Autodesk Inventor part; units mm, degrees
(part 2 of 3)
sketch "Sketch8" plane through (0, 0, 9) normal (0, 0, -1) x (-1, 0, 0)
  circle A0 centre (-7.891, 75.5745) radius 2.55 projected
  circle A1 centre (-45.291, 75.5745) radius 2.55 projected
  circle A2 centre (-26.591, 75.5745) radius 2.55 projected
  arc A3 (-14.3665, 90.3518) -> (-12.2661, 92.5181) centre (-15.59, 93.6395) ccw projected
  arc A4 (-14.955, 86.1645) -> (-14.3665, 90.3518) centre (-14.955, 88.2995) ccw projected
  line L0 (-17.86, 86.1645) -> (-14.955, 86.1645) projected
  line L1 (-17.86, 86.6645) -> (-17.86, 86.1645) projected
  line L2 (-14.955, 86.6645) -> (-17.86, 86.6645) projected
  arc A5 (-14.955, 86.6645) -> (-14.955, 89.9345) centre (-14.955, 88.2995) ccw projected
  line L3 (-16.225, 89.9345) -> (-14.955, 89.9345) projected
  arc A6 (-16.7766, 90.8841) -> (-16.225, 89.9345) centre (-16.225, 90.5695) ccw projected
  arc A7 (-16.7766, 90.8841) -> (-12.6611, 92.9903) centre (-15.59, 93.6395) ccw projected
  arc A8 (-12.6611, 92.9903) -> (-11.1978, 95.4421) centre (-12.6138, 94.6246) ccw projected
  line L4 (-11.8328, 96.5419) -> (-11.1978, 95.4421) projected
  arc A9 (-10.733, 97.1769) -> (-11.8328, 96.5419) centre (-11.2829, 96.8594) ccw projected
  line L5 (-9.2805, 94.6611) -> (-10.733, 97.1769) projected
  line L6 (-9.7135, 94.4111) -> (-9.2805, 94.6611) projected
  line L7 (-11.157, 93.0638) -> (-9.7135, 94.4111) projected
  arc A10 (-12.2661, 92.5181) -> (-11.157, 93.0638) centre (-12.6138, 94.6246) ccw projected
  arc A11 (-19.049, 94.2238) -> (-18.2231, 91.3216) centre (-15.59, 93.6395) ccw projected
  arc A12 (-22.3811, 96.8271) -> (-19.049, 94.2238) centre (-20.5321, 95.7596) ccw projected
  line L8 (-20.9286, 99.3429) -> (-22.3811, 96.8271) projected
  line L9 (-20.4955, 99.0929) -> (-20.9286, 99.3429) projected
  line L10 (-21.948, 96.5771) -> (-20.4955, 99.0929) projected
  arc A13 (-21.948, 96.5771) -> (-19.1161, 94.9421) centre (-20.5321, 95.7596) ccw projected
  line L11 (-18.4811, 96.0419) -> (-19.1161, 94.9421) projected
  arc A14 (-17.3829, 96.0448) -> (-18.4811, 96.0419) centre (-17.9312, 95.7244) ccw projected
  arc A15 (-17.3829, 96.0448) -> (-17.6167, 91.4276) centre (-15.59, 93.6395) ccw projected
  arc A16 (-17.6167, 91.4276) -> (-16.225, 88.9345) centre (-16.225, 90.5695) ccw projected
  line L12 (-14.955, 88.9345) -> (-16.225, 88.9345) projected
  arc A17 (-14.955, 87.6645) -> (-14.955, 88.9345) centre (-14.955, 88.2995) ccw projected
  line L13 (-17.86, 87.6645) -> (-14.955, 87.6645) projected
  line L14 (-17.86, 88.1645) -> (-17.86, 87.6645) projected
  line L15 (-18.3051, 90.0883) -> (-17.86, 88.1645) projected
  arc A18 (-18.2231, 91.3216) -> (-18.3051, 90.0883) centre (-16.225, 90.5695) ccw projected
  arc A19 (-13.3545, 96.3429) -> (-16.2808, 97.0788) centre (-15.59, 93.6395) ccw projected
  arc A20 (-9.4339, 97.9269) -> (-13.3545, 96.3429) centre (-11.2829, 96.8594) ccw projected
  line L16 (-7.9814, 95.4111) -> (-9.4339, 97.9269) projected
  line L17 (-8.4145, 95.1611) -> (-7.9814, 95.4111) projected
  line L18 (-9.867, 97.6769) -> (-8.4145, 95.1611) projected
  arc A21 (-9.867, 97.6769) -> (-12.6989, 96.0419) centre (-11.2829, 96.8594) ccw projected
  line L19 (-12.0639, 94.9421) -> (-12.6989, 96.0419) projected
  arc A22 (-12.6105, 93.9896) -> (-12.0639, 94.9421) centre (-12.6138, 94.6246) ccw projected
  arc A23 (-12.6105, 93.9896) -> (-16.4922, 96.5006) centre (-15.59, 93.6395) ccw projected
  arc A24 (-16.4922, 96.5006) -> (-19.3472, 96.5419) centre (-17.9312, 95.7244) ccw projected
  line L20 (-19.9822, 95.4421) -> (-19.3472, 96.5419) projected
  arc A25 (-21.082, 96.0771) -> (-19.9822, 95.4421) centre (-20.5321, 95.7596) ccw projected
  line L21 (-19.6295, 98.5929) -> (-21.082, 96.0771) projected
  line L22 (-19.1965, 98.3429) -> (-19.6295, 98.5929) projected
  line L23 (-17.3079, 97.7664) -> (-19.1965, 98.3429) projected
  arc A26 (-16.2808, 97.0788) -> (-17.3079, 97.7664) centre (-17.9312, 95.7244) ccw projected
  arc A27 (-33.0665, 90.3518) -> (-30.9661, 92.5181) centre (-34.29, 93.6395) ccw projected
  arc A28 (-33.655, 86.1645) -> (-33.0665, 90.3518) centre (-33.655, 88.2995) ccw projected
  line L24 (-36.56, 86.1645) -> (-33.655, 86.1645) projected
  line L25 (-36.56, 86.6645) -> (-36.56, 86.1645) projected
  line L26 (-33.655, 86.6645) -> (-36.56, 86.6645) projected
  arc A29 (-33.655, 86.6645) -> (-33.655, 89.9345) centre (-33.655, 88.2995) ccw projected
  line L27 (-34.925, 89.9345) -> (-33.655, 89.9345) projected
  arc A30 (-35.4766, 90.8841) -> (-34.925, 89.9345) centre (-34.925, 90.5695) ccw projected
  arc A31 (-35.4766, 90.8841) -> (-31.3611, 92.9903) centre (-34.29, 93.6395) ccw projected
  arc A32 (-31.3611, 92.9903) -> (-29.8978, 95.4421) centre (-31.3138, 94.6246) ccw projected
  line L28 (-30.5328, 96.5419) -> (-29.8978, 95.4421) projected
  arc A33 (-29.433, 97.1769) -> (-30.5328, 96.5419) centre (-29.9829, 96.8594) ccw projected
  line L29 (-27.9805, 94.6611) -> (-29.433, 97.1769) projected
  line L30 (-28.4135, 94.4111) -> (-27.9805, 94.6611) projected
  line L31 (-29.857, 93.0638) -> (-28.4135, 94.4111) projected
  arc A34 (-30.9661, 92.5181) -> (-29.857, 93.0638) centre (-31.3138, 94.6246) ccw projected
  arc A35 (-37.749, 94.2238) -> (-36.9231, 91.3216) centre (-34.29, 93.6395) ccw projected
  arc A36 (-41.0811, 96.8271) -> (-37.749, 94.2238) centre (-39.2321, 95.7596) ccw projected
  line L32 (-39.6286, 99.3429) -> (-41.0811, 96.8271) projected
  line L33 (-39.1955, 99.0929) -> (-39.6286, 99.3429) projected
  line L34 (-40.648, 96.5771) -> (-39.1955, 99.0929) projected
  arc A37 (-40.648, 96.5771) -> (-37.8161, 94.9421) centre (-39.2321, 95.7596) ccw projected
  line L35 (-37.1811, 96.0419) -> (-37.8161, 94.9421) projected
  arc A38 (-36.0829, 96.0448) -> (-37.1811, 96.0419) centre (-36.6312, 95.7244) ccw projected
  arc A39 (-36.0829, 96.0448) -> (-36.3167, 91.4276) centre (-34.29, 93.6395) ccw projected
  arc A40 (-36.3167, 91.4276) -> (-34.925, 88.9345) centre (-34.925, 90.5695) ccw projected
  line L36 (-33.655, 88.9345) -> (-34.925, 88.9345) projected
  arc A41 (-33.655, 87.6645) -> (-33.655, 88.9345) centre (-33.655, 88.2995) ccw projected
  line L37 (-36.56, 87.6645) -> (-33.655, 87.6645) projected
  line L38 (-36.56, 88.1645) -> (-36.56, 87.6645) projected
  line L39 (-37.0051, 90.0883) -> (-36.56, 88.1645) projected
  arc A42 (-36.9231, 91.3216) -> (-37.0051, 90.0883) centre (-34.925, 90.5695) ccw projected
  arc A43 (-32.0545, 96.3429) -> (-34.9808, 97.0788) centre (-34.29, 93.6395) ccw projected
  arc A44 (-28.1339, 97.9269) -> (-32.0545, 96.3429) centre (-29.9829, 96.8594) ccw projected
  line L40 (-26.6814, 95.4111) -> (-28.1339, 97.9269) projected
  line L41 (-27.1145, 95.1611) -> (-26.6814, 95.4111) projected
  line L42 (-28.567, 97.6769) -> (-27.1145, 95.1611) projected
  arc A45 (-28.567, 97.6769) -> (-31.3989, 96.0419) centre (-29.9829, 96.8594) ccw projected
  line L43 (-30.7639, 94.9421) -> (-31.3989, 96.0419) projected
  arc A46 (-31.3105, 93.9896) -> (-30.7639, 94.9421) centre (-31.3138, 94.6246) ccw projected
  arc A47 (-31.3105, 93.9896) -> (-35.1922, 96.5006) centre (-34.29, 93.6395) ccw projected
  arc A48 (-35.1922, 96.5006) -> (-38.0472, 96.5419) centre (-36.6312, 95.7244) ccw projected
  line L44 (-38.6822, 95.4421) -> (-38.0472, 96.5419) projected
  arc A49 (-39.782, 96.0771) -> (-38.6822, 95.4421) centre (-39.2321, 95.7596) ccw projected
  line L45 (-38.3295, 98.5929) -> (-39.782, 96.0771) projected
  line L46 (-37.8965, 98.3429) -> (-38.3295, 98.5929) projected
  line L47 (-36.0079, 97.7664) -> (-37.8965, 98.3429) projected
  arc A50 (-34.9808, 97.0788) -> (-36.0079, 97.7664) centre (-36.6312, 95.7244) ccw projected
  arc A51 (-51.7665, 90.3518) -> (-49.6661, 92.5181) centre (-52.99, 93.6395) ccw projected
  arc A52 (-52.355, 86.1645) -> (-51.7665, 90.3518) centre (-52.355, 88.2995) ccw projected
  line L48 (-55.26, 86.1645) -> (-52.355, 86.1645) projected
  line L49 (-55.26, 86.6645) -> (-55.26, 86.1645) projected
  line L50 (-52.355, 86.6645) -> (-55.26, 86.6645) projected
  arc A53 (-52.355, 86.6645) -> (-52.355, 89.9345) centre (-52.355, 88.2995) ccw projected
  line L51 (-53.625, 89.9345) -> (-52.355, 89.9345) projected
  arc A54 (-54.1766, 90.8841) -> (-53.625, 89.9345) centre (-53.625, 90.5695) ccw projected
  arc A55 (-54.1766, 90.8841) -> (-50.0611, 92.9903) centre (-52.99, 93.6395) ccw projected
  arc A56 (-50.0611, 92.9903) -> (-48.5978, 95.4421) centre (-50.0138, 94.6246) ccw projected
  line L52 (-49.2328, 96.5419) -> (-48.5978, 95.4421) projected
  arc A57 (-48.133, 97.1769) -> (-49.2328, 96.5419) centre (-48.6829, 96.8594) ccw projected
  line L53 (-46.6805, 94.6611) -> (-48.133, 97.1769) projected
  line L54 (-47.1135, 94.4111) -> (-46.6805, 94.6611) projected
  line L55 (-48.557, 93.0638) -> (-47.1135, 94.4111) projected
  arc A58 (-49.6661, 92.5181) -> (-48.557, 93.0638) centre (-50.0138, 94.6246) ccw projected
  arc A59 (-56.449, 94.2238) -> (-55.6231, 91.3216) centre (-52.99, 93.6395) ccw projected
  arc A60 (-59.7811, 96.8271) -> (-56.449, 94.2238) centre (-57.9321, 95.7596) ccw projected
  line L56 (-58.3286, 99.3429) -> (-59.7811, 96.8271) projected
  line L57 (-57.8955, 99.0929) -> (-58.3286, 99.3429) projected
  line L58 (-59.348, 96.5771) -> (-57.8955, 99.0929) projected
  arc A61 (-59.348, 96.5771) -> (-56.5161, 94.9421) centre (-57.9321, 95.7596) ccw projected
  line L59 (-55.8811, 96.0419) -> (-56.5161, 94.9421) projected
  arc A62 (-54.7829, 96.0448) -> (-55.8811, 96.0419) centre (-55.3312, 95.7244) ccw projected
  arc A63 (-54.7829, 96.0448) -> (-55.0167, 91.4276) centre (-52.99, 93.6395) ccw projected
  arc A64 (-55.0167, 91.4276) -> (-53.625, 88.9345) centre (-53.625, 90.5695) ccw projected
  line L60 (-52.355, 88.9345) -> (-53.625, 88.9345) projected
  arc A65 (-52.355, 87.6645) -> (-52.355, 88.9345) centre (-52.355, 88.2995) ccw projected
  line L61 (-55.26, 87.6645) -> (-52.355, 87.6645) projected
  line L62 (-55.26, 88.1645) -> (-55.26, 87.6645) projected
  line L63 (-55.7051, 90.0883) -> (-55.26, 88.1645) projected
  arc A66 (-55.6231, 91.3216) -> (-55.7051, 90.0883) centre (-53.625, 90.5695) ccw projected
  arc A67 (-50.7545, 96.3429) -> (-53.6808, 97.0788) centre (-52.99, 93.6395) ccw projected
  arc A68 (-46.8339, 97.9269) -> (-50.7545, 96.3429) centre (-48.6829, 96.8594) ccw projected
  line L64 (-45.3814, 95.4111) -> (-46.8339, 97.9269) projected
  line L65 (-45.8145, 95.1611) -> (-45.3814, 95.4111) projected
  line L66 (-47.267, 97.6769) -> (-45.8145, 95.1611) projected
  arc A69 (-47.267, 97.6769) -> (-50.0989, 96.0419) centre (-48.6829, 96.8594) ccw projected
  line L67 (-49.4639, 94.9421) -> (-50.0989, 96.0419) projected
  arc A70 (-50.0105, 93.9896) -> (-49.4639, 94.9421) centre (-50.0138, 94.6246) ccw projected
  arc A71 (-50.0105, 93.9896) -> (-53.8922, 96.5006) centre (-52.99, 93.6395) ccw projected
  arc A72 (-53.8922, 96.5006) -> (-56.7472, 96.5419) centre (-55.3312, 95.7244) ccw projected
  line L68 (-57.3822, 95.4421) -> (-56.7472, 96.5419) projected
  arc A73 (-58.482, 96.0771) -> (-57.3822, 95.4421) centre (-57.9321, 95.7596) ccw projected
  line L69 (-57.0295, 98.5929) -> (-58.482, 96.0771) projected
  line L70 (-56.5965, 98.3429) -> (-57.0295, 98.5929) projected
  line L71 (-54.7079, 97.7664) -> (-56.5965, 98.3429) projected
  arc A74 (-53.6808, 97.0788) -> (-54.7079, 97.7664) centre (-55.3312, 95.7244) ccw projected
  arc A75 (-14.3665, 76.7318) -> (-12.2661, 78.8981) centre (-15.59, 80.0195) ccw projected
  arc A76 (-14.955, 72.5445) -> (-14.3665, 76.7318) centre (-14.955, 74.6795) ccw projected
  line L72 (-17.86, 72.5445) -> (-14.955, 72.5445) projected
  line L73 (-17.86, 73.0445) -> (-17.86, 72.5445) projected
  line L74 (-14.955, 73.0445) -> (-17.86, 73.0445) projected
  arc A77 (-14.955, 73.0445) -> (-14.955, 76.3145) centre (-14.955, 74.6795) ccw projected
  line L75 (-16.225, 76.3145) -> (-14.955, 76.3145) projected
  arc A78 (-16.7766, 77.2641) -> (-16.225, 76.3145) centre (-16.225, 76.9495) ccw projected
  arc A79 (-16.7766, 77.2641) -> (-12.6611, 79.3703) centre (-15.59, 80.0195) ccw projected
  arc A80 (-12.6611, 79.3703) -> (-11.1978, 81.8221) centre (-12.6138, 81.0046) ccw projected
  line L76 (-11.8328, 82.9219) -> (-11.1978, 81.8221) projected
  arc A81 (-10.733, 83.5569) -> (-11.8328, 82.9219) centre (-11.2829, 83.2394) ccw projected
  line L77 (-9.2805, 81.0411) -> (-10.733, 83.5569) projected
  line L78 (-9.7135, 80.7911) -> (-9.2805, 81.0411) projected
  line L79 (-11.157, 79.4438) -> (-9.7135, 80.7911) projected
  arc A82 (-12.2661, 78.8981) -> (-11.157, 79.4438) centre (-12.6138, 81.0046) ccw projected
  arc A83 (-19.049, 80.6038) -> (-18.2231, 77.7016) centre (-15.59, 80.0195) ccw projected
  arc A84 (-22.3811, 83.2071) -> (-19.049, 80.6038) centre (-20.5321, 82.1396) ccw projected
  line L80 (-20.9286, 85.7229) -> (-22.3811, 83.2071) projected
  line L81 (-20.4955, 85.4729) -> (-20.9286, 85.7229) projected
  line L82 (-21.948, 82.9571) -> (-20.4955, 85.4729) projected
  arc A85 (-21.948, 82.9571) -> (-19.1161, 81.3221) centre (-20.5321, 82.1396) ccw projected
  line L83 (-18.4811, 82.4219) -> (-19.1161, 81.3221) projected
  arc A86 (-17.3829, 82.4248) -> (-18.4811, 82.4219) centre (-17.9312, 82.1044) ccw projected
  arc A87 (-17.3829, 82.4248) -> (-17.6167, 77.8076) centre (-15.59, 80.0195) ccw projected
  arc A88 (-17.6167, 77.8076) -> (-16.225, 75.3145) centre (-16.225, 76.9495) ccw projected
  line L84 (-14.955, 75.3145) -> (-16.225, 75.3145) projected
  arc A89 (-14.955, 74.0445) -> (-14.955, 75.3145) centre (-14.955, 74.6795) ccw projected
  line L85 (-17.86, 74.0445) -> (-14.955, 74.0445) projected
  line L86 (-17.86, 74.5445) -> (-17.86, 74.0445) projected
  line L87 (-18.3051, 76.4683) -> (-17.86, 74.5445) projected
  arc A90 (-18.2231, 77.7016) -> (-18.3051, 76.4683) centre (-16.225, 76.9495) ccw projected
  arc A91 (-13.3545, 82.7229) -> (-16.2808, 83.4588) centre (-15.59, 80.0195) ccw projected
  arc A92 (-9.4339, 84.3069) -> (-13.3545, 82.7229) centre (-11.2829, 83.2394) ccw projected
  line L88 (-7.9814, 81.7911) -> (-9.4339, 84.3069) projected
  line L89 (-8.4145, 81.5411) -> (-7.9814, 81.7911) projected
  line L90 (-9.867, 84.0569) -> (-8.4145, 81.5411) projected
  arc A93 (-9.867, 84.0569) -> (-12.6989, 82.4219) centre (-11.2829, 83.2394) ccw projected
  line L91 (-12.0639, 81.3221) -> (-12.6989, 82.4219) projected
  arc A94 (-12.6105, 80.3696) -> (-12.0639, 81.3221) centre (-12.6138, 81.0046) ccw projected
  arc A95 (-12.6105, 80.3696) -> (-16.4922, 82.8806) centre (-15.59, 80.0195) ccw projected
  arc A96 (-16.4922, 82.8806) -> (-19.3472, 82.9219) centre (-17.9312, 82.1044) ccw projected
  line L92 (-19.9822, 81.8221) -> (-19.3472, 82.9219) projected
  arc A97 (-21.082, 82.4571) -> (-19.9822, 81.8221) centre (-20.5321, 82.1396) ccw projected
  line L93 (-19.6295, 84.9729) -> (-21.082, 82.4571) projected
  line L94 (-19.1965, 84.7229) -> (-19.6295, 84.9729) projected
  line L95 (-17.3079, 84.1464) -> (-19.1965, 84.7229) projected
  arc A98 (-16.2808, 83.4588) -> (-17.3079, 84.1464) centre (-17.9312, 82.1044) ccw projected
  arc A99 (-33.0665, 76.7318) -> (-30.9661, 78.8981) centre (-34.29, 80.0195) ccw projected
  arc A100 (-33.655, 72.5445) -> (-33.0665, 76.7318) centre (-33.655, 74.6795) ccw projected
  line L96 (-36.56, 72.5445) -> (-33.655, 72.5445) projected
  line L97 (-36.56, 73.0445) -> (-36.56, 72.5445) projected
  line L98 (-33.655, 73.0445) -> (-36.56, 73.0445) projected
  arc A101 (-33.655, 73.0445) -> (-33.655, 76.3145) centre (-33.655, 74.6795) ccw projected
  line L99 (-34.925, 76.3145) -> (-33.655, 76.3145) projected
  arc A102 (-35.4766, 77.2641) -> (-34.925, 76.3145) centre (-34.925, 76.9495) ccw projected
  arc A103 (-35.4766, 77.2641) -> (-31.3611, 79.3703) centre (-34.29, 80.0195) ccw projected
  arc A104 (-31.3611, 79.3703) -> (-29.8978, 81.8221) centre (-31.3138, 81.0046) ccw projected
  line L100 (-30.5328, 82.9219) -> (-29.8978, 81.8221) projected
  arc A105 (-29.433, 83.5569) -> (-30.5328, 82.9219) centre (-29.9829, 83.2394) ccw projected
  line L101 (-27.9805, 81.0411) -> (-29.433, 83.5569) projected
  line L102 (-28.4135, 80.7911) -> (-27.9805, 81.0411) projected
  line L103 (-29.857, 79.4438) -> (-28.4135, 80.7911) projected
  arc A106 (-30.9661, 78.8981) -> (-29.857, 79.4438) centre (-31.3138, 81.0046) ccw projected
  arc A107 (-37.749, 80.6038) -> (-36.9231, 77.7016) centre (-34.29, 80.0195) ccw projected
  arc A108 (-41.0811, 83.2071) -> (-37.749, 80.6038) centre (-39.2321, 82.1396) ccw projected
  line L104 (-39.6286, 85.7229) -> (-41.0811, 83.2071) projected
  line L105 (-39.1955, 85.4729) -> (-39.6286, 85.7229) projected
  line L106 (-40.648, 82.9571) -> (-39.1955, 85.4729) projected
  arc A109 (-40.648, 82.9571) -> (-37.8161, 81.3221) centre (-39.2321, 82.1396) ccw projected
  line L107 (-37.1811, 82.4219) -> (-37.8161, 81.3221) projected
  arc A110 (-36.0829, 82.4248) -> (-37.1811, 82.4219) centre (-36.6312, 82.1044) ccw projected
  arc A111 (-36.0829, 82.4248) -> (-36.3167, 77.8076) centre (-34.29, 80.0195) ccw projected
  arc A112 (-36.3167, 77.8076) -> (-34.925, 75.3145) centre (-34.925, 76.9495) ccw projected
  line L108 (-33.655, 75.3145) -> (-34.925, 75.3145) projected
  arc A113 (-33.655, 74.0445) -> (-33.655, 75.3145) centre (-33.655, 74.6795) ccw projected
  line L109 (-36.56, 74.0445) -> (-33.655, 74.0445) projected
  line L110 (-36.56, 74.5445) -> (-36.56, 74.0445) projected
  line L111 (-37.0051, 76.4683) -> (-36.56, 74.5445) projected
  arc A114 (-36.9231, 77.7016) -> (-37.0051, 76.4683) centre (-34.925, 76.9495) ccw projected
  arc A115 (-32.0545, 82.7229) -> (-34.9808, 83.4588) centre (-34.29, 80.0195) ccw projected
  arc A116 (-28.1339, 84.3069) -> (-32.0545, 82.7229) centre (-29.9829, 83.2394) ccw projected
  line L112 (-26.6814, 81.7911) -> (-28.1339, 84.3069) projected
  line L113 (-27.1145, 81.5411) -> (-26.6814, 81.7911) projected
  line L114 (-28.567, 84.0569) -> (-27.1145, 81.5411) projected
  arc A117 (-28.567, 84.0569) -> (-31.3989, 82.4219) centre (-29.9829, 83.2394) ccw projected
  line L115 (-30.7639, 81.3221) -> (-31.3989, 82.4219) projected
  arc A118 (-31.3105, 80.3696) -> (-30.7639, 81.3221) centre (-31.3138, 81.0046) ccw projected
  arc A119 (-31.3105, 80.3696) -> (-35.1922, 82.8806) centre (-34.29, 80.0195) ccw projected
  arc A120 (-35.1922, 82.8806) -> (-38.0472, 82.9219) centre (-36.6312, 82.1044) ccw projected
  line L116 (-38.6822, 81.8221) -> (-38.0472, 82.9219) projected
  arc A121 (-39.782, 82.4571) -> (-38.6822, 81.8221) centre (-39.2321, 82.1396) ccw projected
  line L117 (-38.3295, 84.9729) -> (-39.782, 82.4571) projected
  line L118 (-37.8965, 84.7229) -> (-38.3295, 84.9729) projected
  line L119 (-36.0079, 84.1464) -> (-37.8965, 84.7229) projected
  arc A122 (-34.9808, 83.4588) -> (-36.0079, 84.1464) centre (-36.6312, 82.1044) ccw projected
  arc A123 (-56.449, 80.6038) -> (-55.6231, 77.7016) centre (-52.99, 80.0195) ccw projected
  arc A124 (-59.7811, 83.2071) -> (-56.449, 80.6038) centre (-57.9321, 82.1396) ccw projected
  line L120 (-58.3286, 85.7229) -> (-59.7811, 83.2071) projected
  line L121 (-57.8955, 85.4729) -> (-58.3286, 85.7229) projected
  line L122 (-59.348, 82.9571) -> (-57.8955, 85.4729) projected
  arc A125 (-59.348, 82.9571) -> (-56.5161, 81.3221) centre (-57.9321, 82.1396) ccw projected
  line L123 (-55.8811, 82.4219) -> (-56.5161, 81.3221) projected
  arc A126 (-54.7829, 82.4248) -> (-55.8811, 82.4219) centre (-55.3312, 82.1044) ccw projected
  arc A127 (-54.7829, 82.4248) -> (-55.0167, 77.8076) centre (-52.99, 80.0195) ccw projected
  arc A128 (-55.0167, 77.8076) -> (-53.625, 75.3145) centre (-53.625, 76.9495) ccw projected
  line L124 (-52.355, 75.3145) -> (-53.625, 75.3145) projected
  arc A129 (-52.355, 74.0445) -> (-52.355, 75.3145) centre (-52.355, 74.6795) ccw projected
  line L125 (-55.26, 74.0445) -> (-52.355, 74.0445) projected
  line L126 (-55.26, 74.5445) -> (-55.26, 74.0445) projected
  line L127 (-55.7051, 76.4683) -> (-55.26, 74.5445) projected
  arc A130 (-55.6231, 77.7016) -> (-55.7051, 76.4683) centre (-53.625, 76.9495) ccw projected
  arc A131 (-50.0105, 80.3696) -> (-53.8922, 82.8806) centre (-52.99, 80.0195) ccw projected
  arc A132 (-53.8922, 82.8806) -> (-56.7472, 82.9219) centre (-55.3312, 82.1044) ccw projected
  line L128 (-57.3822, 81.8221) -> (-56.7472, 82.9219) projected
  arc A133 (-58.482, 82.4571) -> (-57.3822, 81.8221) centre (-57.9321, 82.1396) ccw projected
  line L129 (-57.0295, 84.9729) -> (-58.482, 82.4571) projected
  line L130 (-56.5965, 84.7229) -> (-57.0295, 84.9729) projected
  line L131 (-54.7079, 84.1464) -> (-56.5965, 84.7229) projected
  arc A134 (-53.6808, 83.4588) -> (-54.7079, 84.1464) centre (-55.3312, 82.1044) ccw projected
  arc A135 (-50.7545, 82.7229) -> (-53.6808, 83.4588) centre (-52.99, 80.0195) ccw projected
  arc A136 (-46.8339, 84.3069) -> (-50.7545, 82.7229) centre (-48.6829, 83.2394) ccw projected
  line L132 (-45.3814, 81.7911) -> (-46.8339, 84.3069) projected
  line L133 (-45.8145, 81.5411) -> (-45.3814, 81.7911) projected
  line L134 (-47.267, 84.0569) -> (-45.8145, 81.5411) projected
  arc A137 (-47.267, 84.0569) -> (-50.0989, 82.4219) centre (-48.6829, 83.2394) ccw projected
  line L135 (-49.4639, 81.3221) -> (-50.0989, 82.4219) projected
  arc A138 (-50.0105, 80.3696) -> (-49.4639, 81.3221) centre (-50.0138, 81.0046) ccw projected
  arc A139 (-50.0611, 79.3703) -> (-48.5978, 81.8221) centre (-50.0138, 81.0046) ccw projected
  line L136 (-49.2328, 82.9219) -> (-48.5978, 81.8221) projected
  arc A140 (-48.133, 83.5569) -> (-49.2328, 82.9219) centre (-48.6829, 83.2394) ccw projected
  line L137 (-46.6805, 81.0411) -> (-48.133, 83.5569) projected
  line L138 (-47.1135, 80.7911) -> (-46.6805, 81.0411) projected
  line L139 (-48.557, 79.4438) -> (-47.1135, 80.7911) projected
  arc A141 (-49.6661, 78.8981) -> (-48.557, 79.4438) centre (-50.0138, 81.0046) ccw projected
  arc A142 (-51.7665, 76.7318) -> (-49.6661, 78.8981) centre (-52.99, 80.0195) ccw projected
  arc A143 (-52.355, 72.5445) -> (-51.7665, 76.7318) centre (-52.355, 74.6795) ccw projected
  line L140 (-55.26, 72.5445) -> (-52.355, 72.5445) projected
  line L141 (-55.26, 73.0445) -> (-55.26, 72.5445) projected
  line L142 (-52.355, 73.0445) -> (-55.26, 73.0445) projected
  arc A144 (-52.355, 73.0445) -> (-52.355, 76.3145) centre (-52.355, 74.6795) ccw projected
  line L143 (-53.625, 76.3145) -> (-52.355, 76.3145) projected
  arc A145 (-54.1766, 77.2641) -> (-53.625, 76.3145) centre (-53.625, 76.9495) ccw projected
  arc A146 (-54.1766, 77.2641) -> (-50.0611, 79.3703) centre (-52.99, 80.0195) ccw projected
  line L144 (-2, 65.9374) -> (-66.58, 65.9374) projected
  line L145 (-2, 105.95) -> (-2, 65.9374) projected
  line L146 (-66.58, 105.95) -> (-2, 105.95) projected
  line L147 (-66.58, 65.9374) -> (-66.58, 105.95) projected
  line L148 (-9.7135, 80.7911) -> (-9.2805, 81.0411) projected
  line L149 (-9.2805, 81.0411) -> (-8.4145, 81.5411)
  line L150 (-17.86, 73.0445) -> (-17.86, 72.5445) projected
  line L151 (-17.86, 74.0445) -> (-17.86, 73.0445)
  line L152 (-20.4955, 85.4729) -> (-20.9286, 85.7229) projected
  line L153 (-20.4955, 85.4729) -> (-19.6295, 84.9729)
  line L154 (-8.4145, 95.1611) -> (-7.9814, 95.4111) projected
  line L155 (-8.4145, 95.1611) -> (-9.2805, 94.6611)
  line L156 (-17.86, 86.6645) -> (-17.86, 86.1645) projected
  line L157 (-17.86, 87.6645) -> (-17.86, 86.6645)
  line L158 (-20.4955, 99.0929) -> (-19.6295, 98.5929)
  line L159 (-27.1145, 95.1611) -> (-26.6814, 95.4111) projected
  line L160 (-27.1145, 95.1611) -> (-27.9805, 94.6611)
  line L161 (-27.1145, 81.5411) -> (-27.9805, 81.0411)
  line L162 (-36.56, 73.0445) -> (-36.56, 72.5445) projected
  line L163 (-36.56, 74.0445) -> (-36.56, 73.0445)
  line L164 (-40.648, 82.9571) -> (-39.1955, 85.4729) projected
  line L165 (-38.3295, 84.9729) -> (-39.1955, 85.4729)
  line L166 (-33.655, 86.6645) -> (-36.56, 86.6645) projected
  line L167 (-36.56, 86.6645) -> (-36.56, 87.6645)
  line L168 (-40.648, 96.5771) -> (-39.1955, 99.0929) projected
  line L169 (-39.1955, 99.0929) -> (-38.3295, 98.5929)
  line L170 (-46.6805, 81.0411) -> (-45.8145, 81.5411)
  line L171 (-55.26, 73.0445) -> (-55.26, 72.5445) projected
  line L172 (-55.26, 73.0445) -> (-55.26, 74.0445)
  line L173 (-57.8955, 85.4729) -> (-57.0295, 84.9729)
  line L174 (-55.26, 87.6645) -> (-55.26, 86.6645)
  line L175 (-45.8145, 95.1611) -> (-45.3814, 95.4111) projected
  line L176 (-45.8145, 95.1611) -> (-46.6805, 94.6611)
  line L177 (-59.348, 96.5771) -> (-57.8955, 99.0929) projected
  line L178 (-57.0295, 98.5929) -> (-58.482, 96.0771) projected
  line L179 (-57.8955, 99.0929) -> (-57.0295, 98.5929)
  line L180 (-37.34, 83.0695) -> (-31.24, 83.0695)
  line L181 (-31.24, 83.0695) -> (-31.24, 76.9695)
  line L182 (-31.24, 76.9695) -> (-37.34, 76.9695)
  line L183 (-37.34, 76.9695) -> (-37.34, 83.0695)
  line L184 (-37.34, 83.0695) -> (-31.24, 76.9695) construction
  line L185 (-31.24, 83.0695) -> (-37.34, 76.9695) construction
  line L186 (-37.34, 96.6895) -> (-31.24, 96.6895)
  line L187 (-31.24, 96.6895) -> (-31.24, 90.5895)
  line L188 (-31.24, 90.5895) -> (-37.34, 90.5895)
  line L189 (-37.34, 90.5895) -> (-37.34, 96.6895)
  line L190 (-37.34, 96.6895) -> (-31.24, 90.5895) construction
  line L191 (-31.24, 96.6895) -> (-37.34, 90.5895) construction
  line L192 (-12.54, 96.6895) -> (-18.64, 96.6895)
  line L193 (-18.64, 96.6895) -> (-18.64, 90.5895)
  line L194 (-18.64, 90.5895) -> (-12.54, 90.5895)
  line L195 (-12.54, 90.5895) -> (-12.54, 96.6895)
  line L196 (-12.54, 96.6895) -> (-18.64, 90.5895) construction
  line L197 (-18.64, 96.6895) -> (-12.54, 90.5895) construction
  line L198 (-12.54, 83.0695) -> (-18.64, 83.0695)
  line L199 (-18.64, 83.0695) -> (-18.64, 76.9695)
  line L200 (-18.64, 76.9695) -> (-12.54, 76.9695)
  line L201 (-12.54, 76.9695) -> (-12.54, 83.0695)
  line L202 (-12.54, 83.0695) -> (-18.64, 76.9695) construction
  line L203 (-18.64, 83.0695) -> (-12.54, 76.9695) construction
  line L204 (-49.94, 83.0695) -> (-56.04, 83.0695)
  line L205 (-56.04, 83.0695) -> (-56.04, 76.9695)
  line L206 (-56.04, 76.9695) -> (-49.94, 76.9695)
  line L207 (-49.94, 76.9695) -> (-49.94, 83.0695)
  line L208 (-49.94, 83.0695) -> (-56.04, 76.9695) construction
  line L209 (-56.04, 83.0695) -> (-49.94, 76.9695) construction
  line L210 (-49.94, 96.6895) -> (-56.04, 96.6895)
  line L211 (-56.04, 96.6895) -> (-56.04, 90.5895)
  line L212 (-56.04, 90.5895) -> (-49.94, 90.5895)
  line L213 (-49.94, 90.5895) -> (-49.94, 96.6895)
  line L214 (-49.94, 96.6895) -> (-56.04, 90.5895) construction
  line L215 (-56.04, 96.6895) -> (-49.94, 90.5895) construction
  point P0 (0, 0)
  point P1 (-37.0599, 90.5895)
  point P2 (-37.34, 91.9064)
  point P3 (-32.5569, 96.6895)
  point P4 (-32.1111, 96.6895)
  point P5 (-31.24, 91.9064)
  point P6 (-32.5569, 90.5895)
  point P7 (-37.0599, 76.9695)
  point P8 (-37.34, 78.2864)
  point P9 (-32.5569, 83.0695)
  point P10 (-32.1111, 83.0695)
  point P11 (-31.24, 78.2864)
  point P12 (-32.5569, 76.9695)
  point P13 (-51.2569, 83.0695)
  point P14 (-50.8111, 83.0695)
  point P15 (-49.94, 78.2864)
  point P16 (-51.2569, 76.9695)
  point P17 (-55.7599, 76.9695)
  point P18 (-56.04, 78.2864)
  point P19 (-18.3599, 76.9695)
  point P20 (-18.64, 78.2864)
  point P21 (-13.8569, 83.0695)
  point P22 (-13.4111, 83.0695)
  point P23 (-12.54, 78.2864)
  point P24 (-13.8569, 76.9695)
  point P25 (-55.7599, 90.5895)
  point P26 (-56.04, 91.9064)
  point P27 (-51.2569, 96.6895)
  point P28 (-50.8111, 96.6895)
  point P29 (-49.94, 91.9064)
  point P30 (-51.2569, 90.5895)
  point P31 (-18.3599, 90.5895)
  point P32 (-18.64, 91.9064)
  point P33 (-13.8569, 96.6895)
  point P34 (-13.4111, 96.6895)
  point P35 (-12.54, 91.9064)
  point P36 (-13.8569, 90.5895)
  dimension "d82" = 6.1
  dimension "d83" = 6.1
  constraints: 108 end point, 12 midpoint, 12 parallel, 10 equal length, 8 perpendicular, 6 horizontal, 4 vertical, 3 collinear, 1 point on line
  measures "d82" distance of L194.end L193.end
  measures "d83" distance of L193.end L192.end
extrude "Extrusion10" add sketch "Sketch8" along normal blind 3.5
fillet "Fillet1" radius 5 8 edges at (68.58, 107.95, 5) (0, 107.95, 5) (0, 0, 5) (68.58, 0, 5) (66.58, 105.95, 2.75) (2, 105.95, 2.75) (2, 65.9374, 2.75) (66.58, 65.9374, 2.75)
chamfer "Chamfer1" distance 2 angle 45 8 edges at (34.29, 0, 10) (67.1155, 1.4645, 10) (68.58, 53.975, 10) (67.1155, 106.4855, 10) (34.29, 107.95, 10) (1.4645, 106.4855, 10) (0, 53.975, 10) (1.4645, 1.4645, 10)
sketch "Sketch9" plane through (34.29, 35.56, 4) normal (0, 0, 1) x (1, 0, 0)
  line L0 (0, 25.4139) -> (22.0091, -12.707) construction
  line L1 (22.0091, -12.707) -> (-22.0091, -12.707) construction
  line L2 (-22.0091, -12.707) -> (0, 25.4139) construction
  circle A0 centre (0, 25.4139) radius 2
  circle A1 centre (22.0091, -12.707) radius 2
  circle A2 centre (-22.0091, -12.707) radius 2
  circle A3 centre (0, 0) radius 21.3606 projected
  point P0 (-34.29, -35.56)
  dimension "d94" = 44.0182
  dimension "d95" = 4
  constraints: 6 end point, 4 coincident, 3 centre point, 2 equal radius, 1 horizontal, 7 other
  measures "d94" distance of L0.start L0.end
  measures "d95" diameter of A2
extrude "Extrusion11" cut sketch "Sketch9" against normal through all contours A0 | A1 | A2
sketch "Sketch10" plane through (0, 0, 10) normal (0, 0, 1) x (1, 0, 0)
  arc A0 (17.6167, 91.4276) -> (17.3829, 96.0448) centre (15.59, 93.6395) ccw projected
  arc A1 (18.4811, 96.0419) -> (17.3829, 96.0448) centre (17.9312, 95.7244) ccw projected
  line L0 (18.4811, 96.0419) -> (19.1161, 94.9421) projected
  arc A2 (19.1161, 94.9421) -> (21.948, 96.5771) centre (20.5321, 95.7596) ccw projected
  line L1 (21.948, 96.5771) -> (20.4955, 99.0929) projected
  line L2 (20.4955, 99.0929) -> (20.9286, 99.3429) projected
  line L3 (20.9286, 99.3429) -> (22.3811, 96.8271) projected
  arc A3 (19.049, 94.2238) -> (22.3811, 96.8271) centre (20.5321, 95.7596) ccw projected
  arc A4 (18.2231, 91.3216) -> (19.049, 94.2238) centre (15.59, 93.6395) ccw projected
  arc A5 (18.3051, 90.0883) -> (18.2231, 91.3216) centre (16.225, 90.5695) ccw projected
  line L4 (18.3051, 90.0883) -> (17.86, 88.1645) projected
  line L5 (17.86, 88.1645) -> (17.86, 87.6645) projected
  line L6 (17.86, 87.6645) -> (14.955, 87.6645) projected
  arc A6 (14.955, 88.9345) -> (14.955, 87.6645) centre (14.955, 88.2995) ccw projected
  line L7 (14.955, 88.9345) -> (16.225, 88.9345) projected
  arc A7 (16.225, 88.9345) -> (17.6167, 91.4276) centre (16.225, 90.5695) ccw projected
  arc A8 (16.2808, 97.0788) -> (13.3545, 96.3429) centre (15.59, 93.6395) ccw projected
  arc A9 (17.3079, 97.7664) -> (16.2808, 97.0788) centre (17.9312, 95.7244) ccw projected
  line L8 (17.3079, 97.7664) -> (19.1965, 98.3429) projected
  line L9 (19.1965, 98.3429) -> (19.6295, 98.5929) projected
  line L10 (19.6295, 98.5929) -> (21.082, 96.0771) projected
  arc A10 (19.9822, 95.4421) -> (21.082, 96.0771) centre (20.5321, 95.7596) ccw projected
  line L11 (19.9822, 95.4421) -> (19.3472, 96.5419) projected
  arc A11 (19.3472, 96.5419) -> (16.4922, 96.5006) centre (17.9312, 95.7244) ccw projected
  arc A12 (16.4922, 96.5006) -> (12.6105, 93.9896) centre (15.59, 93.6395) ccw projected
  arc A13 (12.0639, 94.9421) -> (12.6105, 93.9896) centre (12.6138, 94.6246) ccw projected
  line L12 (12.0639, 94.9421) -> (12.6989, 96.0419) projected
  arc A14 (12.6989, 96.0419) -> (9.867, 97.6769) centre (11.2829, 96.8594) ccw projected
  line L13 (9.867, 97.6769) -> (8.4145, 95.1611) projected
  line L14 (8.4145, 95.1611) -> (7.9814, 95.4111) projected
  line L15 (7.9814, 95.4111) -> (9.4339, 97.9269) projected
  arc A15 (13.3545, 96.3429) -> (9.4339, 97.9269) centre (11.2829, 96.8594) ccw projected
  arc A16 (12.6611, 92.9903) -> (16.7766, 90.8841) centre (15.59, 93.6395) ccw projected
  arc A17 (16.225, 89.9345) -> (16.7766, 90.8841) centre (16.225, 90.5695) ccw projected
  line L16 (16.225, 89.9345) -> (14.955, 89.9345) projected
  arc A18 (14.955, 89.9345) -> (14.955, 86.6645) centre (14.955, 88.2995) ccw projected
  line L17 (14.955, 86.6645) -> (17.86, 86.6645) projected
  line L18 (17.86, 86.6645) -> (17.86, 86.1645) projected
  line L19 (17.86, 86.1645) -> (14.955, 86.1645) projected
  arc A19 (14.3665, 90.3518) -> (14.955, 86.1645) centre (14.955, 88.2995) ccw projected
  arc A20 (12.2661, 92.5181) -> (14.3665, 90.3518) centre (15.59, 93.6395) ccw projected
  arc A21 (11.157, 93.0638) -> (12.2661, 92.5181) centre (12.6138, 94.6246) ccw projected
  line L20 (11.157, 93.0638) -> (9.7135, 94.4111) projected
  line L21 (9.7135, 94.4111) -> (9.2805, 94.6611) projected
  line L22 (9.2805, 94.6611) -> (10.733, 97.1769) projected
  arc A22 (11.8328, 96.5419) -> (10.733, 97.1769) centre (11.2829, 96.8594) ccw projected
  line L23 (11.8328, 96.5419) -> (11.1978, 95.4421) projected
  arc A23 (11.1978, 95.4421) -> (12.6611, 92.9903) centre (12.6138, 94.6246) ccw projected
  arc A24 (36.3167, 91.4276) -> (36.0829, 96.0448) centre (34.29, 93.6395) ccw projected
  arc A25 (37.1811, 96.0419) -> (36.0829, 96.0448) centre (36.6312, 95.7244) ccw projected
  line L24 (37.1811, 96.0419) -> (37.8161, 94.9421) projected
  arc A26 (37.8161, 94.9421) -> (40.648, 96.5771) centre (39.2321, 95.7596) ccw projected
  line L25 (40.648, 96.5771) -> (39.1955, 99.0929) projected
  line L26 (39.1955, 99.0929) -> (39.6286, 99.3429) projected
  line L27 (39.6286, 99.3429) -> (41.0811, 96.8271) projected
  arc A27 (37.749, 94.2238) -> (41.0811, 96.8271) centre (39.2321, 95.7596) ccw projected
  arc A28 (36.9231, 91.3216) -> (37.749, 94.2238) centre (34.29, 93.6395) ccw projected
  arc A29 (37.0051, 90.0883) -> (36.9231, 91.3216) centre (34.925, 90.5695) ccw projected
  line L28 (37.0051, 90.0883) -> (36.56, 88.1645) projected
  line L29 (36.56, 88.1645) -> (36.56, 87.6645) projected
  line L30 (36.56, 87.6645) -> (33.655, 87.6645) projected
  arc A30 (33.655, 88.9345) -> (33.655, 87.6645) centre (33.655, 88.2995) ccw projected
  line L31 (33.655, 88.9345) -> (34.925, 88.9345) projected
  arc A31 (34.925, 88.9345) -> (36.3167, 91.4276) centre (34.925, 90.5695) ccw projected
  arc A32 (34.9808, 97.0788) -> (32.0545, 96.3429) centre (34.29, 93.6395) ccw projected
  arc A33 (36.0079, 97.7664) -> (34.9808, 97.0788) centre (36.6312, 95.7244) ccw projected
  line L32 (36.0079, 97.7664) -> (37.8965, 98.3429) projected
  line L33 (37.8965, 98.3429) -> (38.3295, 98.5929) projected
  line L34 (38.3295, 98.5929) -> (39.782, 96.0771) projected
  arc A34 (38.6822, 95.4421) -> (39.782, 96.0771) centre (39.2321, 95.7596) ccw projected
  line L35 (38.6822, 95.4421) -> (38.0472, 96.5419) projected
  arc A35 (38.0472, 96.5419) -> (35.1922, 96.5006) centre (36.6312, 95.7244) ccw projected
  arc A36 (35.1922, 96.5006) -> (31.3105, 93.9896) centre (34.29, 93.6395) ccw projected
  arc A37 (30.7639, 94.9421) -> (31.3105, 93.9896) centre (31.3138, 94.6246) ccw projected
  line L36 (30.7639, 94.9421) -> (31.3989, 96.0419) projected
  arc A38 (31.3989, 96.0419) -> (28.567, 97.6769) centre (29.9829, 96.8594) ccw projected
  line L37 (28.567, 97.6769) -> (27.1145, 95.1611) projected
  line L38 (27.1145, 95.1611) -> (26.6814, 95.4111) projected
  line L39 (26.6814, 95.4111) -> (28.1339, 97.9269) projected
  arc A39 (32.0545, 96.3429) -> (28.1339, 97.9269) centre (29.9829, 96.8594) ccw projected
  arc A40 (31.3611, 92.9903) -> (35.4766, 90.8841) centre (34.29, 93.6395) ccw projected
  arc A41 (34.925, 89.9345) -> (35.4766, 90.8841) centre (34.925, 90.5695) ccw projected
  line L40 (34.925, 89.9345) -> (33.655, 89.9345) projected
  arc A42 (33.655, 89.9345) -> (33.655, 86.6645) centre (33.655, 88.2995) ccw projected
  line L41 (33.655, 86.6645) -> (36.56, 86.6645) projected
  line L42 (36.56, 86.6645) -> (36.56, 86.1645) projected
  line L43 (36.56, 86.1645) -> (33.655, 86.1645) projected
  arc A43 (33.0665, 90.3518) -> (33.655, 86.1645) centre (33.655, 88.2995) ccw projected
  arc A44 (30.9661, 92.5181) -> (33.0665, 90.3518) centre (34.29, 93.6395) ccw projected
  arc A45 (29.857, 93.0638) -> (30.9661, 92.5181) centre (31.3138, 94.6246) ccw projected
  line L44 (29.857, 93.0638) -> (28.4135, 94.4111) projected
  line L45 (28.4135, 94.4111) -> (27.9805, 94.6611) projected
  line L46 (27.9805, 94.6611) -> (29.433, 97.1769) projected
  arc A46 (30.5328, 96.5419) -> (29.433, 97.1769) centre (29.9829, 96.8594) ccw projected
  line L47 (30.5328, 96.5419) -> (29.8978, 95.4421) projected
  arc A47 (29.8978, 95.4421) -> (31.3611, 92.9903) centre (31.3138, 94.6246) ccw projected
  arc A48 (55.0167, 91.4276) -> (54.7829, 96.0448) centre (52.99, 93.6395) ccw projected
  arc A49 (55.8811, 96.0419) -> (54.7829, 96.0448) centre (55.3312, 95.7244) ccw projected
  line L48 (55.8811, 96.0419) -> (56.5161, 94.9421) projected
  arc A50 (56.5161, 94.9421) -> (59.348, 96.5771) centre (57.9321, 95.7596) ccw projected
  line L49 (59.348, 96.5771) -> (57.8955, 99.0929) projected
  line L50 (57.8955, 99.0929) -> (58.3286, 99.3429) projected
  line L51 (58.3286, 99.3429) -> (59.7811, 96.8271) projected
  arc A51 (56.449, 94.2238) -> (59.7811, 96.8271) centre (57.9321, 95.7596) ccw projected
  arc A52 (55.6231, 91.3216) -> (56.449, 94.2238) centre (52.99, 93.6395) ccw projected
  arc A53 (55.7051, 90.0883) -> (55.6231, 91.3216) centre (53.625, 90.5695) ccw projected
  line L52 (55.7051, 90.0883) -> (55.26, 88.1645) projected
  line L53 (55.26, 88.1645) -> (55.26, 87.6645) projected
  line L54 (55.26, 87.6645) -> (52.355, 87.6645) projected
  arc A54 (52.355, 88.9345) -> (52.355, 87.6645) centre (52.355, 88.2995) ccw projected
  line L55 (52.355, 88.9345) -> (53.625, 88.9345) projected
  arc A55 (53.625, 88.9345) -> (55.0167, 91.4276) centre (53.625, 90.5695) ccw projected
  arc A56 (53.6808, 97.0788) -> (50.7545, 96.3429) centre (52.99, 93.6395) ccw projected
  arc A57 (54.7079, 97.7664) -> (53.6808, 97.0788) centre (55.3312, 95.7244) ccw projected
  line L56 (54.7079, 97.7664) -> (56.5965, 98.3429) projected
  line L57 (56.5965, 98.3429) -> (57.0295, 98.5929) projected
  line L58 (57.0295, 98.5929) -> (58.482, 96.0771) projected
  arc A58 (57.3822, 95.4421) -> (58.482, 96.0771) centre (57.9321, 95.7596) ccw projected
  line L59 (57.3822, 95.4421) -> (56.7472, 96.5419) projected
  arc A59 (56.7472, 96.5419) -> (53.8922, 96.5006) centre (55.3312, 95.7244) ccw projected
  arc A60 (53.8922, 96.5006) -> (50.0105, 93.9896) centre (52.99, 93.6395) ccw projected
  arc A61 (49.4639, 94.9421) -> (50.0105, 93.9896) centre (50.0138, 94.6246) ccw projected
  line L60 (49.4639, 94.9421) -> (50.0989, 96.0419) projected
  arc A62 (50.0989, 96.0419) -> (47.267, 97.6769) centre (48.6829, 96.8594) ccw projected
  line L61 (47.267, 97.6769) -> (45.8145, 95.1611) projected
  line L62 (45.8145, 95.1611) -> (45.3814, 95.4111) projected
  line L63 (45.3814, 95.4111) -> (46.8339, 97.9269) projected
  arc A63 (50.7545, 96.3429) -> (46.8339, 97.9269) centre (48.6829, 96.8594) ccw projected
  arc A64 (50.0611, 92.9903) -> (54.1766, 90.8841) centre (52.99, 93.6395) ccw projected
  arc A65 (53.625, 89.9345) -> (54.1766, 90.8841) centre (53.625, 90.5695) ccw projected
  line L64 (53.625, 89.9345) -> (52.355, 89.9345) projected
  arc A66 (52.355, 89.9345) -> (52.355, 86.6645) centre (52.355, 88.2995) ccw projected
  line L65 (52.355, 86.6645) -> (55.26, 86.6645) projected
  line L66 (55.26, 86.6645) -> (55.26, 86.1645) projected
  line L67 (55.26, 86.1645) -> (52.355, 86.1645) projected
  arc A67 (51.7665, 90.3518) -> (52.355, 86.1645) centre (52.355, 88.2995) ccw projected
  arc A68 (49.6661, 92.5181) -> (51.7665, 90.3518) centre (52.99, 93.6395) ccw projected
  arc A69 (48.557, 93.0638) -> (49.6661, 92.5181) centre (50.0138, 94.6246) ccw projected
  line L68 (48.557, 93.0638) -> (47.1135, 94.4111) projected
  line L69 (47.1135, 94.4111) -> (46.6805, 94.6611) projected
  line L70 (46.6805, 94.6611) -> (48.133, 97.1769) projected
  arc A70 (49.2328, 96.5419) -> (48.133, 97.1769) centre (48.6829, 96.8594) ccw projected
  line L71 (49.2328, 96.5419) -> (48.5978, 95.4421) projected
  arc A71 (48.5978, 95.4421) -> (50.0611, 92.9903) centre (50.0138, 94.6246) ccw projected
  arc A72 (17.6167, 77.8076) -> (17.3829, 82.4248) centre (15.59, 80.0195) ccw projected
  arc A73 (18.4811, 82.4219) -> (17.3829, 82.4248) centre (17.9312, 82.1044) ccw projected
  line L72 (18.4811, 82.4219) -> (19.1161, 81.3221) projected
  arc A74 (19.1161, 81.3221) -> (21.948, 82.9571) centre (20.5321, 82.1396) ccw projected
  line L73 (21.948, 82.9571) -> (20.4955, 85.4729) projected
  line L74 (20.4955, 85.4729) -> (20.9286, 85.7229) projected
  line L75 (20.9286, 85.7229) -> (22.3811, 83.2071) projected
  arc A75 (19.049, 80.6038) -> (22.3811, 83.2071) centre (20.5321, 82.1396) ccw projected
  arc A76 (18.2231, 77.7016) -> (19.049, 80.6038) centre (15.59, 80.0195) ccw projected
  arc A77 (18.3051, 76.4683) -> (18.2231, 77.7016) centre (16.225, 76.9495) ccw projected
  line L76 (18.3051, 76.4683) -> (17.86, 74.5445) projected
  line L77 (17.86, 74.5445) -> (17.86, 74.0445) projected
  line L78 (17.86, 74.0445) -> (14.955, 74.0445) projected
  arc A78 (14.955, 75.3145) -> (14.955, 74.0445) centre (14.955, 74.6795) ccw projected
  line L79 (14.955, 75.3145) -> (16.225, 75.3145) projected
  arc A79 (16.225, 75.3145) -> (17.6167, 77.8076) centre (16.225, 76.9495) ccw projected
  arc A80 (16.2808, 83.4588) -> (13.3545, 82.7229) centre (15.59, 80.0195) ccw projected
  arc A81 (17.3079, 84.1464) -> (16.2808, 83.4588) centre (17.9312, 82.1044) ccw projected
  line L80 (17.3079, 84.1464) -> (19.1965, 84.7229) projected
  line L81 (19.1965, 84.7229) -> (19.6295, 84.9729) projected
  line L82 (19.6295, 84.9729) -> (21.082, 82.4571) projected
  arc A82 (19.9822, 81.8221) -> (21.082, 82.4571) centre (20.5321, 82.1396) ccw projected
  line L83 (19.9822, 81.8221) -> (19.3472, 82.9219) projected
  arc A83 (19.3472, 82.9219) -> (16.4922, 82.8806) centre (17.9312, 82.1044) ccw projected
  arc A84 (16.4922, 82.8806) -> (12.6105, 80.3696) centre (15.59, 80.0195) ccw projected
  arc A85 (12.0639, 81.3221) -> (12.6105, 80.3696) centre (12.6138, 81.0046) ccw projected
  line L84 (12.0639, 81.3221) -> (12.6989, 82.4219) projected
  arc A86 (12.6989, 82.4219) -> (9.867, 84.0569) centre (11.2829, 83.2394) ccw projected
  line L85 (9.867, 84.0569) -> (8.4145, 81.5411) projected
  line L86 (8.4145, 81.5411) -> (7.9814, 81.7911) projected
  line L87 (7.9814, 81.7911) -> (9.4339, 84.3069) projected
  arc A87 (13.3545, 82.7229) -> (9.4339, 84.3069) centre (11.2829, 83.2394) ccw projected
  arc A88 (12.6611, 79.3703) -> (16.7766, 77.2641) centre (15.59, 80.0195) ccw projected
  arc A89 (16.225, 76.3145) -> (16.7766, 77.2641) centre (16.225, 76.9495) ccw projected
  line L88 (16.225, 76.3145) -> (14.955, 76.3145) projected
  arc A90 (14.955, 76.3145) -> (14.955, 73.0445) centre (14.955, 74.6795) ccw projected
  line L89 (14.955, 73.0445) -> (17.86, 73.0445) projected
  line L90 (17.86, 73.0445) -> (17.86, 72.5445) projected
  line L91 (17.86, 72.5445) -> (14.955, 72.5445) projected
  arc A91 (14.3665, 76.7318) -> (14.955, 72.5445) centre (14.955, 74.6795) ccw projected
  arc A92 (12.2661, 78.8981) -> (14.3665, 76.7318) centre (15.59, 80.0195) ccw projected
  arc A93 (11.157, 79.4438) -> (12.2661, 78.8981) centre (12.6138, 81.0046) ccw projected
  line L92 (11.157, 79.4438) -> (9.7135, 80.7911) projected
  line L93 (9.7135, 80.7911) -> (9.2805, 81.0411) projected
  line L94 (9.2805, 81.0411) -> (10.733, 83.5569) projected
  arc A94 (11.8328, 82.9219) -> (10.733, 83.5569) centre (11.2829, 83.2394) ccw projected
  line L95 (11.8328, 82.9219) -> (11.1978, 81.8221) projected
  arc A95 (11.1978, 81.8221) -> (12.6611, 79.3703) centre (12.6138, 81.0046) ccw projected
  arc A96 (36.3167, 77.8076) -> (36.0829, 82.4248) centre (34.29, 80.0195) ccw projected
  arc A97 (37.1811, 82.4219) -> (36.0829, 82.4248) centre (36.6312, 82.1044) ccw projected
  line L96 (37.1811, 82.4219) -> (37.8161, 81.3221) projected
  arc A98 (37.8161, 81.3221) -> (40.648, 82.9571) centre (39.2321, 82.1396) ccw projected
  line L97 (40.648, 82.9571) -> (39.1955, 85.4729) projected
  line L98 (39.1955, 85.4729) -> (39.6286, 85.7229) projected
  line L99 (39.6286, 85.7229) -> (41.0811, 83.2071) projected
  arc A99 (37.749, 80.6038) -> (41.0811, 83.2071) centre (39.2321, 82.1396) ccw projected
  arc A100 (36.9231, 77.7016) -> (37.749, 80.6038) centre (34.29, 80.0195) ccw projected
  arc A101 (37.0051, 76.4683) -> (36.9231, 77.7016) centre (34.925, 76.9495) ccw projected
  line L100 (37.0051, 76.4683) -> (36.56, 74.5445) projected
  line L101 (36.56, 74.5445) -> (36.56, 74.0445) projected
  line L102 (36.56, 74.0445) -> (33.655, 74.0445) projected
  arc A102 (33.655, 75.3145) -> (33.655, 74.0445) centre (33.655, 74.6795) ccw projected
  line L103 (33.655, 75.3145) -> (34.925, 75.3145) projected
  arc A103 (34.925, 75.3145) -> (36.3167, 77.8076) centre (34.925, 76.9495) ccw projected
  arc A104 (34.9808, 83.4588) -> (32.0545, 82.7229) centre (34.29, 80.0195) ccw projected
  arc A105 (36.0079, 84.1464) -> (34.9808, 83.4588) centre (36.6312, 82.1044) ccw projected
  line L104 (36.0079, 84.1464) -> (37.8965, 84.7229) projected
  line L105 (37.8965, 84.7229) -> (38.3295, 84.9729) projected
  line L106 (38.3295, 84.9729) -> (39.782, 82.4571) projected
  arc A106 (38.6822, 81.8221) -> (39.782, 82.4571) centre (39.2321, 82.1396) ccw projected
  line L107 (38.6822, 81.8221) -> (38.0472, 82.9219) projected
  arc A107 (38.0472, 82.9219) -> (35.1922, 82.8806) centre (36.6312, 82.1044) ccw projected
  arc A108 (35.1922, 82.8806) -> (31.3105, 80.3696) centre (34.29, 80.0195) ccw projected
  arc A109 (30.7639, 81.3221) -> (31.3105, 80.3696) centre (31.3138, 81.0046) ccw projected
  line L108 (30.7639, 81.3221) -> (31.3989, 82.4219) projected
  arc A110 (31.3989, 82.4219) -> (28.567, 84.0569) centre (29.9829, 83.2394) ccw projected
  line L109 (28.567, 84.0569) -> (27.1145, 81.5411) projected
  line L110 (27.1145, 81.5411) -> (26.6814, 81.7911) projected
  line L111 (26.6814, 81.7911) -> (28.1339, 84.3069) projected
  arc A111 (32.0545, 82.7229) -> (28.1339, 84.3069) centre (29.9829, 83.2394) ccw projected
  arc A112 (31.3611, 79.3703) -> (35.4766, 77.2641) centre (34.29, 80.0195) ccw projected
  arc A113 (34.925, 76.3145) -> (35.4766, 77.2641) centre (34.925, 76.9495) ccw projected
  line L112 (34.925, 76.3145) -> (33.655, 76.3145) projected
  arc A114 (33.655, 76.3145) -> (33.655, 73.0445) centre (33.655, 74.6795) ccw projected
  line L113 (33.655, 73.0445) -> (36.56, 73.0445) projected
  line L114 (36.56, 73.0445) -> (36.56, 72.5445) projected
  line L115 (36.56, 72.5445) -> (33.655, 72.5445) projected
  arc A115 (33.0665, 76.7318) -> (33.655, 72.5445) centre (33.655, 74.6795) ccw projected
  arc A116 (30.9661, 78.8981) -> (33.0665, 76.7318) centre (34.29, 80.0195) ccw projected
  arc A117 (29.857, 79.4438) -> (30.9661, 78.8981) centre (31.3138, 81.0046) ccw projected
  line L116 (29.857, 79.4438) -> (28.4135, 80.7911) projected
  line L117 (28.4135, 80.7911) -> (27.9805, 81.0411) projected
  line L118 (27.9805, 81.0411) -> (29.433, 83.5569) projected
  arc A118 (30.5328, 82.9219) -> (29.433, 83.5569) centre (29.9829, 83.2394) ccw projected
  line L119 (30.5328, 82.9219) -> (29.8978, 81.8221) projected
  arc A119 (29.8978, 81.8221) -> (31.3611, 79.3703) centre (31.3138, 81.0046) ccw projected
  arc A120 (49.6661, 78.8981) -> (51.7665, 76.7318) centre (52.99, 80.0195) ccw projected
  arc A121 (48.557, 79.4438) -> (49.6661, 78.8981) centre (50.0138, 81.0046) ccw projected
  line L120 (48.557, 79.4438) -> (47.1135, 80.7911) projected
  line L121 (47.1135, 80.7911) -> (46.6805, 81.0411) projected
  line L122 (46.6805, 81.0411) -> (48.133, 83.5569) projected
  arc A122 (49.2328, 82.9219) -> (48.133, 83.5569) centre (48.6829, 83.2394) ccw projected
  line L123 (49.2328, 82.9219) -> (48.5978, 81.8221) projected
  arc A123 (48.5978, 81.8221) -> (50.0611, 79.3703) centre (50.0138, 81.0046) ccw projected
  arc A124 (50.0611, 79.3703) -> (54.1766, 77.2641) centre (52.99, 80.0195) ccw projected
  arc A125 (53.625, 76.3145) -> (54.1766, 77.2641) centre (53.625, 76.9495) ccw projected
  line L124 (53.625, 76.3145) -> (52.355, 76.3145) projected
  arc A126 (52.355, 76.3145) -> (52.355, 73.0445) centre (52.355, 74.6795) ccw projected
  line L125 (52.355, 73.0445) -> (55.26, 73.0445) projected
  line L126 (55.26, 73.0445) -> (55.26, 72.5445) projected
  line L127 (55.26, 72.5445) -> (52.355, 72.5445) projected
  arc A127 (51.7665, 76.7318) -> (52.355, 72.5445) centre (52.355, 74.6795) ccw projected
  arc A128 (55.6231, 77.7016) -> (56.449, 80.6038) centre (52.99, 80.0195) ccw projected
  arc A129 (55.7051, 76.4683) -> (55.6231, 77.7016) centre (53.625, 76.9495) ccw projected
  line L128 (55.7051, 76.4683) -> (55.26, 74.5445) projected
  line L129 (55.26, 74.5445) -> (55.26, 74.0445) projected
  line L130 (55.26, 74.0445) -> (52.355, 74.0445) projected
  arc A130 (52.355, 75.3145) -> (52.355, 74.0445) centre (52.355, 74.6795) ccw projected
  line L131 (52.355, 75.3145) -> (53.625, 75.3145) projected
  arc A131 (53.625, 75.3145) -> (55.0167, 77.8076) centre (53.625, 76.9495) ccw projected
  arc A132 (55.0167, 77.8076) -> (54.7829, 82.4248) centre (52.99, 80.0195) ccw projected
  arc A133 (55.8811, 82.4219) -> (54.7829, 82.4248) centre (55.3312, 82.1044) ccw projected
  line L132 (55.8811, 82.4219) -> (56.5161, 81.3221) projected
  arc A134 (56.5161, 81.3221) -> (59.348, 82.9571) centre (57.9321, 82.1396) ccw projected
  line L133 (59.348, 82.9571) -> (57.8955, 85.4729) projected
  line L134 (57.8955, 85.4729) -> (58.3286, 85.7229) projected
  line L135 (58.3286, 85.7229) -> (59.7811, 83.2071) projected
  arc A135 (56.449, 80.6038) -> (59.7811, 83.2071) centre (57.9321, 82.1396) ccw projected
  arc A136 (53.6808, 83.4588) -> (50.7545, 82.7229) centre (52.99, 80.0195) ccw projected
  arc A137 (54.7079, 84.1464) -> (53.6808, 83.4588) centre (55.3312, 82.1044) ccw projected
  line L136 (54.7079, 84.1464) -> (56.5965, 84.7229) projected
  line L137 (56.5965, 84.7229) -> (57.0295, 84.9729) projected
  line L138 (57.0295, 84.9729) -> (58.482, 82.4571) projected
  arc A138 (57.3822, 81.8221) -> (58.482, 82.4571) centre (57.9321, 82.1396) ccw projected
  line L139 (57.3822, 81.8221) -> (56.7472, 82.9219) projected
  arc A139 (56.7472, 82.9219) -> (53.8922, 82.8806) centre (55.3312, 82.1044) ccw projected
  arc A140 (53.8922, 82.8806) -> (50.0105, 80.3696) centre (52.99, 80.0195) ccw projected
  arc A141 (49.4639, 81.3221) -> (50.0105, 80.3696) centre (50.0138, 81.0046) ccw projected
  line L140 (49.4639, 81.3221) -> (50.0989, 82.4219) projected
  arc A142 (50.0989, 82.4219) -> (47.267, 84.0569) centre (48.6829, 83.2394) ccw projected
  line L141 (47.267, 84.0569) -> (45.8145, 81.5411) projected
  line L142 (45.8145, 81.5411) -> (45.3814, 81.7911) projected
  line L143 (45.3814, 81.7911) -> (46.8339, 84.3069) projected
  arc A143 (50.7545, 82.7229) -> (46.8339, 84.3069) centre (48.6829, 83.2394) ccw projected
  circle A144 centre (34.29, 35.56) radius 30.149 projected
  circle A145 centre (26.591, 75.5745) radius 2.55 projected
  circle A146 centre (45.291, 75.5745) radius 2.55 projected
  circle A147 centre (7.891, 75.5745) radius 2.55 projected
  line L144 (51.7673, 70.964) -> (51.7673, 71.5445) projected
  line L145 (51.7673, 71.5445) -> (54.183, 71.5445) projected
  line L146 (54.183, 71.5445) -> (54.183, 70.9739) projected
  line L147 (54.183, 70.9739) -> (52.7776, 69.0769) projected
  line L148 (52.7776, 69.0769) -> (54.1089, 69.0769) projected
  line L149 (54.1089, 69.0769) -> (54.1089, 68.4965) projected
  line L150 (54.1089, 68.4965) -> (51.8489, 68.4965) projected
  line L151 (51.8489, 68.4965) -> (51.8489, 69.0769) projected
  line L152 (51.8489, 69.0769) -> (53.2494, 70.964) projected
  line L153 (53.2494, 70.964) -> (51.7673, 70.964) projected
  line L154 (16.0371, 70.0625) -> (17.0251, 68.4965) projected
  line L155 (17.0251, 68.4965) -> (16.1408, 68.4965) projected
  line L156 (16.1408, 68.4965) -> (15.5529, 69.4672) projected
  line L157 (15.5529, 69.4672) -> (14.9527, 68.4965) projected
  line L158 (14.9527, 68.4965) -> (14.1055, 68.4965) projected
  line L159 (14.1055, 68.4965) -> (15.096, 70.0304) projected
  line L160 (15.096, 70.0304) -> (14.145, 71.5445) projected
  line L161 (14.145, 71.5445) -> (15.0293, 71.5445) projected
  line L162 (15.0293, 71.5445) -> (15.5801, 70.6232) projected
  line L163 (15.5801, 70.6232) -> (16.1458, 71.5445) projected
  line L164 (16.1458, 71.5445) -> (16.993, 71.5445) projected
  line L165 (16.993, 71.5445) -> (16.0371, 70.0625) projected
  line L166 (52.5787, 100.9826) -> (52.5787, 100.4022) projected
  line L167 (52.5787, 100.4022) -> (50.5459, 100.4022) projected
  line L168 (50.5459, 100.4022) -> (50.5459, 103.4502) projected
  line L169 (50.5459, 103.4502) -> (51.3116, 103.4502) projected
  line L170 (51.3116, 103.4502) -> (51.3116, 100.9826) projected
  line L171 (51.3116, 100.9826) -> (52.5787, 100.9826) projected
  line L172 (35.8449, 100.3429) -> (34.8914, 100.3429) projected
  line L173 (34.8914, 100.3429) -> (34.8914, 103.3909) projected
  line L174 (34.8914, 103.3909) -> (35.835, 103.3909) projected
  line L175 (18.4737, 103.4452) -> (18.4737, 100.3972) projected
  line L176 (18.4737, 100.3972) -> (17.713, 100.3972) projected
  line L177 (17.713, 100.3972) -> (17.713, 102.4177) projected
  line L178 (17.713, 102.4177) -> (17.1597, 101.1135) projected
  line L179 (17.1597, 101.1135) -> (16.6361, 101.1135) projected
  line L180 (16.6361, 101.1135) -> (16.0828, 102.4177) projected
  line L181 (16.0828, 102.4177) -> (16.0828, 100.3972) projected
  line L182 (16.0828, 100.3972) -> (15.3615, 100.3972) projected
  line L183 (15.3615, 100.3972) -> (15.3615, 103.4452) projected
  line L184 (15.3615, 103.4452) -> (16.2433, 103.4452) projected
  line L185 (16.2433, 103.4452) -> (16.9201, 101.941) projected
  line L186 (16.9201, 101.941) -> (17.5919, 103.4452) projected
  line L187 (17.5919, 103.4452) -> (18.4737, 103.4452) projected
  line L188 (12.5408, 100.5775) -> (12.5408, 101.3037) projected
  line L189 (12.5408, 101.3037) -> (12.6099, 101.3037) projected
  line L190 (14.8478, 103.2946) -> (14.8478, 102.598) projected
  line L191 (14.8478, 102.598) -> (14.7811, 102.598) projected
  line L192 (34.2591, 103.3909) -> (34.2591, 100.3429) projected
  line L193 (34.2591, 100.3429) -> (33.4984, 100.3429) projected
  line L194 (33.4984, 100.3429) -> (33.4984, 102.3634) projected
  line L195 (33.4984, 102.3634) -> (32.9451, 101.0592) projected
  line L196 (32.9451, 101.0592) -> (32.4214, 101.0592) projected
  line L197 (32.4214, 101.0592) -> (31.8681, 102.3634) projected
  line L198 (31.8681, 102.3634) -> (31.8681, 100.3429) projected
  line L199 (31.8681, 100.3429) -> (31.1469, 100.3429) projected
  line L200 (31.1469, 100.3429) -> (31.1469, 103.3909) projected
  line L201 (31.1469, 103.3909) -> (32.0287, 103.3909) projected
  line L202 (32.0287, 103.3909) -> (32.7055, 101.8866) projected
  line L203 (32.7055, 101.8866) -> (33.3773, 103.3909) projected
  line L204 (33.3773, 103.3909) -> (34.2591, 103.3909) projected
  line L205 (55.2192, 103.5094) -> (55.2192, 103.2402) projected
  line L206 (55.4761, 103.2402) -> (55.4761, 102.5239) projected
  line L207 (54.8314, 100.8986) -> (54.8314, 100.906) projected
  line L208 (54.7474, 100.906) -> (54.7474, 101.5063) projected
  line L209 (54.7474, 101.5063) -> (54.1571, 101.5063) projected
  line L210 (54.1571, 101.5063) -> (54.1571, 102.0768) projected
  line L211 (54.1571, 102.0768) -> (55.4884, 102.0768) projected
  line L212 (34.8519, 71.5445) -> (35.6967, 71.5445) projected
  line L213 (35.6967, 71.5445) -> (34.6444, 69.7685) projected
  line L214 (34.6444, 69.7685) -> (34.6444, 68.4965) projected
  line L215 (34.6444, 68.4965) -> (33.8787, 68.4965) projected
  line L216 (33.8787, 68.4965) -> (33.8787, 69.7315) projected
  line L217 (33.8787, 69.7315) -> (32.8092, 71.5445) projected
  line L218 (32.8092, 71.5445) -> (33.6811, 71.5445) projected
  line L219 (33.6811, 71.5445) -> (34.2764, 70.4577) projected
  line L220 (34.2764, 70.4577) -> (34.8519, 71.5445) projected
  line L221 (63.58, 2) -> (5, 2) projected
  arc A148 (63.58, 2) -> (66.58, 5) centre (63.58, 5) ccw projected
  line L222 (66.58, 102.95) -> (66.58, 5) projected
  arc A149 (66.58, 102.95) -> (63.58, 105.95) centre (63.58, 102.95) ccw projected
  line L223 (5, 105.95) -> (63.58, 105.95) projected
  arc A150 (5, 105.95) -> (2, 102.95) centre (5, 102.95) ccw projected